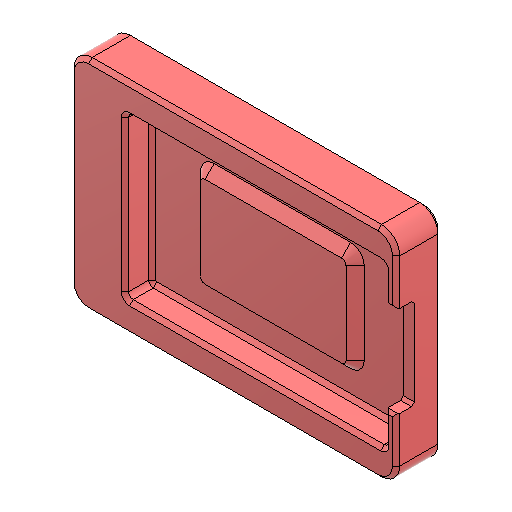
# Autodesk Inventor part: tp4056-pad
Saved by Autodesk Inventor 2026 (Build 300175050, 175E)
## iProperties
Created: 2025-06-22
Part Number: tp4056-pad
Material: ABS Plastic
Document SubType Name: Modeling
Designer: queezz
Density: 1.06 g/cm^3
Appearance: Smooth - Red
Author: queezz
Autodesk Inventor part; units mm, degrees
ref_plane "YZ Plane" through (0, 0, 0) normal (1, 0, 0) x (0, 1, 0)
ref_plane "XZ Plane" through (0, 0, 0) normal (0, 1, 0) x (-1, 0, 0)
ref_plane "XY Plane" through (0, 0, 0) normal (0, 0, 1) x (1, 0, 0)
sketch "Sketch1" plane through (0, 0, 0) normal (0, 0, 1) x (1, 0, 0)
  line L0 (-20.3, 12) -> (15.5, 12)
  line L1 (15.5, 12) -> (15.5, -12)
  line L2 (15.5, -12) -> (-20.3, -12)
  line L3 (-20.3, -12) -> (-20.3, 12)
  line L4 (-14.3, 8.8) -> (14.3, 8.8)
  line L5 (14.3, 8.8) -> (14.3, -8.8)
  line L6 (14.3, -8.8) -> (-14.3, -8.8)
  line L7 (-14.3, -8.8) -> (-14.3, 8.8)
  line L8 (-8, 5) -> (8, 5)
  line L9 (8, 5) -> (8, -5)
  line L10 (8, -5) -> (-8, -5)
  line L11 (-8, -5) -> (-8, 5)
  point P0 (0, 0)
  point P1 (14.3, 0)
  point P2 (0, 8.8)
  point P3 (15.5, 0)
  point P4 (8, 0)
  point P5 (0, 5)
  dimension "d0" = 28.6
  dimension "d1" = 17.6
  dimension "d2" = 1.2
  dimension "d3" = 6
  dimension "d4" = 24
  dimension "d9" = 10
  dimension "d10" = 16
  constraints: 24 end point, 6 parallel, 5 midpoint, 3 horizontal, 3 horizontal alignment, 3 perpendicular, 2 vertical alignment
  measures "d0" distance of L4.start L4.end
  measures "d1" distance of L4.end L5.end
  measures "d2" distance between parallel lines of L1 L5
  measures "d3" distance between parallel lines of L3 L7
  measures "d4" distance of L2.end L0.start
  measures "d9" distance of L8.end L9.end
  measures "d10" distance of L8.start L8.end
extrude "Extrusion1" add sketch "Sketch1" against normal blind 2 contours L0 L1 L2 L3 | L4 L5 L6 L7 | L8 L9 L10 L11
extrude "Extrusion2" add sketch "Sketch1" along normal blind 3 contours L0 L1 L2 L3
extrude "Extrusion3" add sketch "Sketch1" along normal blind 1 contours L8 L9 L10 L11
fillet "Fillet1" radius 2 4 edges at (-20.3, -12, 0.5) (-20.3, 12, 0.5) (15.5, 12, 0.5) (15.5, -12, 0.5)
fillet "Fillet2" radius 0.5 8 edges at (14.3, 8.8, 1.5) (14.3, -8.8, 1.5) (-14.3, 8.8, 1.5) (-14.3, -8.8, 1.5) (-8, 5, 0.5) (-8, -5, 0.5) (8, -5, 0.5) (8, 5, 0.5)
sketch "Sketch2" plane through (15.5, -10, -2) normal (1, 0, 0) x (0, 0, -1)
  line L0 (-5, 0) -> (-5, 20) projected
  line L1 (-5, 5) -> (-3, 5)
  line L2 (-3, 5) -> (-3, 15)
  line L3 (-3, 15) -> (-5, 15)
  line L4 (-5, 15) -> (-5, 5)
  point P0 (-2, 10)
  point P1 (-3, 10)
  dimension "d21" = 10
  dimension "d22" = 2
  constraints: 8 end point, 2 parallel, 1 horizontal, 1 horizontal alignment, 1 midpoint, 1 perpendicular, 1 point on line
  measures "d21" distance of L1.end L2.end
  measures "d22" distance of L2.end L3.end
extrude "Extrusion4" cut sketch "Sketch2" against normal up to surface (1.2 mm away)
chamfer "Chamfer3" distance 0.3 angle 45 4 edges at (14.9, -5, 1) (14.9, -5, 3) (14.9, 5, 1) (14.9, 5, 3)
chamfer "Chamfer1" distance 1 angle 45 8 edges at (-8, 0, 0) (-7.8536, 4.8536, 0) (0, 5, 0) (7.8536, 4.8536, 0) (8, 0, 0) (7.8536, -4.8536, 0) (0, -5, 0) (-7.8536, -4.8536, 0)
chamfer "Chamfer2" distance 0.4 angle 45 34 edges at (0, 8.8, 0) (-14.1536, 8.6536, 0) (-14.3, 0, 0) (-14.1536, -8.6536, 0) (0, -8.8, 0) (14.1536, -8.6536, 0) (14.3, 0, 0) (14.1536, 8.6536, 0) (0, 8.8, 3) (14.1536, 8.6536, 3) (14.3, -6.8, 3) (14.3, 6.8, 3) (14.1536, -8.6536, 3) (0, -8.8, 3) (-14.1536, -8.6536, 3) (-14.3, 0, 3) (-14.1536, 8.6536, 3) (-2.4, 12, 3) (-19.7142, 11.4142, 3) (-20.3, 0, 3) (-19.7142, -11.4142, 3) (-2.4, -12, 3) (14.9142, -11.4142, 3) (15.5, -7.65, 3) (15.5, 7.65, 3) (14.9142, 11.4142, 3) (-20.3, 0, -2) (-19.7142, 11.4142, -2) (-2.4, 12, -2) (14.9142, 11.4142, -2) (15.5, 0, -2) (14.9142, -11.4142, -2) (-2.4, -12, -2) (-19.7142, -11.4142, -2)
body "Solid1"
